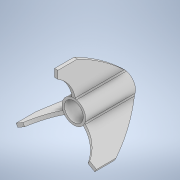
# Autodesk Inventor part: RocketBaseThing
Saved by Autodesk Inventor 2021 (Build 250183000, 183)
## iProperties
Created: 2021-03-21
Part Number: RocketBaseThing
Material: Générique
Document SubType Name: Modeling
Designer: turnb
Density: 1 g/cm^3
Appearance: Par défaut
Author: turnb
Autodesk Inventor part; units mm, degrees
ref_plane "YZ Plane" through (0, 0, 0) normal (1, 0, 0) x (0, 1, 0)
ref_plane "XZ Plane" through (0, 0, 0) normal (0, 1, 0) x (-1, 0, 0)
ref_plane "XY Plane" through (0, 0, 0) normal (0, 0, 1) x (1, 0, 0)
sketch "Esquisse1" plane through (0, 0, 0) normal (0, 0, 1) x (1, 0, 0)
  point P0 (0, 0)
sketch "Esquisse2" plane through (0, 0, 0) normal (0, 0, 1) x (1, 0, 0)
  circle A0 centre (0, 0) radius 17.5
  circle A1 centre (0, 0) radius 14
  dimension "d0" = 35
  dimension "d1" = 28
  constraints: 2 centre point, 2 coincident
  measures "d0" diameter of A0
  measures "d1" diameter of A1
extrude "Extrusion1" add sketch "Esquisse2" along normal blind 74
sketch "Esquisse3" plane through (0, 0, 0) normal (0, 0, -1) x (-1, 0, 0)
  line L0 (2.4577, 17.3266) -> (2.4577, 67.3266)
  line L1 (2.4577, 67.3266) -> (-2.4577, 67.3266)
  line L2 (-2.4577, 67.3266) -> (-2.4577, 17.3266)
  circle A0 centre (0, 0) radius 17.5 projected
  arc A1 (2.4577, 17.3266) -> (-2.4577, 17.3266) centre (0, 0) ccw
  dimension "d4" = 50
  constraints: 6 end point, 4 point on circle, 1 centre point, 1 concentric, 1 parallel
  measures "d4" distance of L0.start L0.end
extrude "Extrusion2" add sketch "Esquisse3" against normal blind 100 contours A0 L2 L1 L0
sketch "Esquisse4" plane through (2.4577, 17.3266, 0) normal (1, 0, 0) x (0, 0, -1)
  point P0 (0, -17.3266)
sketch "Esquisse5" plane through (2.4577, 17.3266, 0) normal (1, 0, 0) x (0, 0, -1)
  point P0 (0, -17.3266)
sketch "Esquisse6" plane through (2.4577, 17.3266, 0) normal (1, 0, 0) x (0, 0, -1)
  line L0 (-74, 0) -> (-74, -34.8266) projected
  line L1 (-100, 0) -> (-100, 50) projected
  arc A0 (-74, 0) -> (-100, 38.4236) centre (-128.4832, -8.8585) ccw
  line L2 (-100, 38.4236) -> (-100, 0)
  line L3 (-74, 0) -> (-100, 0) projected
  line L4 (-74, 0) -> (-100, 0)
  point P0 (0, -17.3266)
  constraints: 4 end point, 2 point on circle, 1 centre point, 1 collinear, 1 point on line, 1 vertical
extrude "Extrusion3" cut sketch "Esquisse6" against normal blind 31
sketch "Esquisse7" plane through (2.4577, 17.3266, 0) normal (1, 0, 0) x (0, 0, -1)
  line L0 (0, 0) -> (0, 50) projected
  line L1 (0, 50) -> (-100, 50) projected
  arc A0 (0, 0) -> (-70.9999, 50) centre (-205.1565, -215.912) ccw
  point P0 (0, -17.3266)
  constraints: 2 point on circle, 1 centre point, 1 point on line
extrude "Extrusion4" cut sketch "Esquisse7" against normal blind 19.75
pattern_circular "Réseau circulaire1" count 3 over 360 about axis through (0, 0, 0) along (0, 0, 1) of "Extrusion2", "Extrusion4", "Extrusion3"
fillet "Congé1" radius 2 6 edges at (-16.2341, -6.5349, 37) (-2.4577, 17.3266, 37) (2.4577, 17.3266, 37) (16.2341, -6.5349, 37) (13.7764, -10.7917, 37) (-13.7764, -10.7917, 37)
